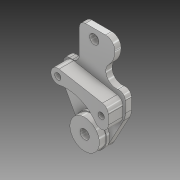
# Autodesk Inventor part: phalanx_2_housing_R
Saved by Autodesk Inventor 2017 SP1 (Build 210196100, 196)
## iProperties
Created: 2017-06-05
Part Number: phalanx_2_housing_R
Material: Generic
Document SubType Name: Modeling
Designer: Tomasz
Density: 1 g/cm^3
Appearance: Aluminum - Polished
Author: Tomasz
Autodesk Inventor part; units mm, degrees
ref_plane "YZ Plane" through (0, 0, 0) normal (1, 0, 0) x (0, 1, 0)
ref_plane "XZ Plane" through (0, 0, 0) normal (0, 1, 0) x (-1, 0, 0)
ref_plane "XY Plane" through (0, 0, 0) normal (0, 0, 1) x (1, 0, 0)
sketch "Sketch1" plane through (0, 0, 0) normal (0, 1, 0) x (-1, 0, 0)
  arc A0 (0, -5) -> (4.4, -2.3749) centre (0, 0) ccw
  line L0 (0, 0) -> (0, 29.6022) construction
  line L1 (10, 9.2633) -> (10, 13.6302)
  line L2 (2.254, 28) -> (-1.8447, 28)
  line L3 (9.4, 6.8883) -> (4.4, -2.3749)
  arc A1 (9.4, 6.8883) -> (10, 9.2633) centre (5, 9.2633) ccw
  arc A2 (-4.4, -2.3749) -> (0, -5) centre (0, 0) ccw
  line L4 (-10, 9.2633) -> (-10, 23)
  line L5 (-5, 28) -> (-1.8447, 28)
  line L6 (-9.4, 6.8883) -> (-4.4, -2.3749)
  arc A3 (-10, 9.2633) -> (-9.4, 6.8883) centre (-5, 9.2633) ccw
  arc A4 (-5, 28) -> (-10, 23) centre (-5, 23) ccw
  arc A5 (4.825, 18) -> (6.95, 15.875) centre (6.95, 18) ccw
  line L7 (4.825, 18) -> (4.825, 28)
  line L8 (4.825, 28) -> (2.254, 28)
  line L9 (10, 13.6302) -> (10, 15.875)
  line L10 (10, 15.875) -> (6.95, 15.875)
  circle A6 centre (0, 0) radius 5
  point P0 (10, 28)
  point P1 (10, 8)
  point P2 (-10, 28)
  dimension "d0" = 10
  dimension "d3" = 10
  dimension "d4" = 28
  dimension "d26" = 8
  dimension "d27" = 5
  dimension "d48" = 5
  dimension "d51" = 3.05
  dimension "d52" = 10
  dimension "d53" = 4.25
  constraints: 22 end point, 12 point on circle, 9 point on line, 7 tangent, 6 centre point, 5 symmetric about line, 4 vertical, 3 coincident, 2 horizontal, 1 perpendicular, 1 vertical alignment, 4 other
  measures "d0" diameter of A0
  measures "d3" distance from line of L1 point (0, 0)
  measures "d4" distance from line of L2 point (0, 0)
  measures "d26" vertical distance of point (10, 8) point (0, 0)
  measures "d27" radius of A1
  measures "d48" radius of A4
  measures "d51" distance from line of A5.centre L1
  measures "d52" distance from line of A5.centre L2
  measures "d53" diameter of A5
extrude "Extrusion1" add sketch "Sketch1" along normal blind 2
sketch "Sketch3" plane through (0, 2, 0) normal (0, 1, 0) x (1, 0, 0)
  line L0 (0, 0) -> (0, -24.7147) construction
  line L1 (-4.825, -28) -> (5, -28) projected
  arc A0 (9.25, -8) -> (4.75, -8) centre (7, -8) ccw
  circle A1 centre (-7, -13.5) radius 2.25
  line L2 (7, -8) -> (7, -11) construction
  line L3 (9.25, -8) -> (9.25, -11)
  line L4 (4.75, -11) -> (4.75, -8)
  arc A2 (9.25, -8) -> (4.75, -8) centre (7, -8) ccw
  arc A3 (4.75, -11) -> (9.25, -11) centre (7, -11) ccw
  arc A4 (-6.5467, -11.2961) -> (5.1678, -6.694) centre (-4.2232, 0) ccw
  line L5 (7.3955, -13.215) -> (-6.6045, -15.715)
  point P0 (-4, -28)
  point P1 (-2.254, -28)
  point P2 (7, -9.5)
  dimension "d28" = 20
  dimension "d29" = 7
  dimension "d46" = 7
  dimension "d47" = 14.5
  dimension "d96" = 4.5
  dimension "d97" = 4.5
  dimension "d136" = 3
  constraints: 12 end point, 12 point on circle, 8 tangent, 5 centre point, 2 coincident, 2 vertical, 1 concentric, 1 horizontal alignment, 1 midpoint, 1 parallel
  measures "d28" distance from line of point (7, -8) L1
  measures "d29" distance from line of point (7, -8) L0
  measures "d46" distance from line of point (-7, -13.5) L0
  measures "d47" distance from line of point (-7, -13.5) L1
  measures "d96" diameter of A0
  measures "d97" diameter of A1
  measures "d136" distance of point (7, -8) L2.end
fillet "Fillet1" radius 2 2 edges at (-10, 1, 15.875) (-4.825, 1, 28)
sketch "Sketch4" plane through (0, 0, 0) normal (0, -1, 0) x (1, 0, 0)
  point P0 (0, 0)
  point P1 (0, 25)
  dimension "d37" = 25
  constraints: 1 vertical alignment
  measures "d37" distance of point (0, 25) point (0, 0)
hole "Hole4" at (0, 0, 25) direction (0, 1, 0) diameter 3 end through all
sketch "Sketch5" plane through (0, 0, 0) normal (0, -1, 0) x (1, 0, 0)
  circle A0 centre (0, 25) radius 1.5 projected
  circle A1 centre (0, 25) radius 1.5 projected
  arc A2 (-2.825, 28) -> (-4.825, 26) centre (-2.825, 26) ccw projected
  line L0 (-4.825, 26) -> (-4.825, 18) projected
  arc A3 (-6.95, 15.875) -> (-4.825, 18) centre (-6.95, 18) ccw projected
  line L1 (-6.95, 15.875) -> (-8, 15.875) projected
  arc A4 (-8, 15.875) -> (-10, 13.875) centre (-8, 13.875) ccw projected
  line L2 (-10, 13.875) -> (-10, 9.2633) projected
  arc A5 (-10, 9.2633) -> (-9.4, 6.8883) centre (-5, 9.2633) ccw projected
  line L3 (-9.4, 6.8883) -> (-4.4, -2.3749) projected
  arc A6 (-4.4, -2.3749) -> (4.4, -2.3749) centre (0, 0) ccw projected
  line L4 (4.4, -2.3749) -> (9.4, 6.8883) projected
  arc A7 (9.4, 6.8883) -> (10, 9.2633) centre (5, 9.2633) ccw projected
  line L5 (10, 9.2633) -> (10, 23) projected
  arc A8 (10, 23) -> (5, 28) centre (5, 23) ccw projected
  line L6 (5, 28) -> (-2.825, 28) projected
  circle A9 centre (0, 25) radius 9.8995 construction
  line L7 (0, 25) -> (17.632, 25) construction
  line L8 (0, 25) -> (13.9609, 10.961) construction
  arc A10 (4.6888, 20.285) -> (10, 16.7785) centre (6.9804, 17.9805) ccw
  arc A11 (4.6888, 20.285) -> (5.9826, 27.9025) centre (0, 25) ccw
  dimension "d55" = 19.799
  dimension "d56" = 45.16
  dimension "d57" = 6.5
  constraints: 5 point on circle, 4 end point, 2 centre point, 2 coincident, 2 point on line, 1 horizontal, 1 midpoint, 3 other
  measures "d56" angle of L7 L8
  measures "d57" diameter of A10
extrude "Extrusion2" cut sketch "Sketch5" against normal through all contours A8 L5 A10 A11
fillet "Fillet2" radius 3 1 edges at (5.9826, 1, 27.9025)
fillet "Fillet3" radius 2 1 edges at (10, 1, 16.7785)
extrude "Extrusion5" add sketch "Sketch3" against normal blind 6.75
sketch "Sketch14" plane through (0, 0, 0) normal (0, -1, 0) x (1, 0, 0)
  circle A0 centre (0, 0) radius 5
  dimension "d123" = 10
  constraints: 1 centre point, 1 coincident
  measures "d123" diameter of A0
extrude "Extrusion6" add sketch "Sketch14" along normal blind 1
sketch "Sketch15" plane through (0, -1, 0) normal (0, -1, 0) x (1, 0, 0)
  circle A0 centre (0, 0) radius 4.75
  dimension "d126" = 9.5
  constraints: 1 centre point, 1 coincident
  measures "d126" diameter of A0
extrude "Extrusion7" add sketch "Sketch15" along normal blind 2.1
sketch "Sketch16" plane through (0, 2, 0) normal (0, 1, 0) x (1, 0, 0)
  point P0 (0, 0)
  point P1 (0, 0)
  constraints: 1 coincident
hole "Hole11" at (0, 2, 0) direction (0, -1, 0) diameter 3 end through all
sketch "Sketch17" plane through (0, -4.75, 0) normal (0, -1, 0) x (1, 0, 0)
  arc A0 (-6.6045, 15.715) -> (-6.5467, 11.2961) centre (-7, 13.5) ccw projected
  arc A1 (5.1678, 6.694) -> (-6.5467, 11.2961) centre (-4.2232, 0) ccw projected
  arc A2 (5.1678, 6.694) -> (9.25, 8) centre (7, 8) ccw projected
  line L0 (9.25, 8) -> (9.25, 11) projected
  arc A3 (9.25, 11) -> (7.3955, 13.215) centre (7, 11) ccw projected
  line L1 (7.3955, 13.215) -> (-6.6045, 15.715) projected
  line L2 (7, 8) -> (7, 11) construction
  point P0 (0, 0)
  point P1 (7, 9.5)
  constraints: 2 end point, 1 midpoint, 1 vertical
hole "mounting" at (7, -4.75, 9.5) at (-7, -4.75, 13.5) direction (0, 1, 0) diameter 2 depth 5.5
body "Solid1"
